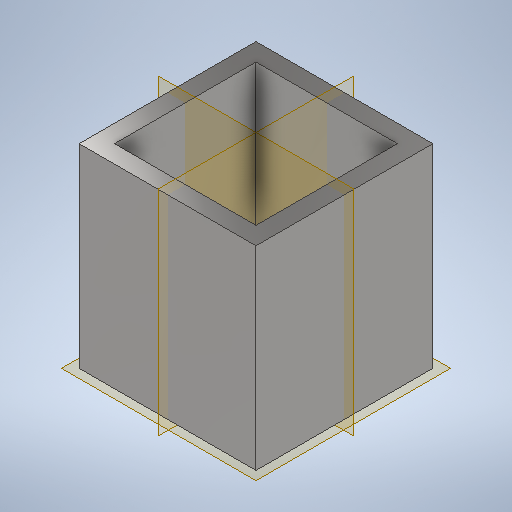
# Autodesk Inventor part: D1_lenght
Saved by Autodesk Inventor 2025.2 (Build 292293000, 293)
## iProperties
Created: 2025-06-19
Part Number: D1_lenght
Material: Steel, Alloy
Document SubType Name: Modeling
Designer: MSIGAMING
Mass: 3061.08 g
Surface Area: 864 cm^2
Volume: 396 cm^3
Density: 7.73 g/cm^3
Appearance: Semi-Polished
Author: MSIGAMING
Autodesk Inventor part; units mm, degrees
sketch "Sketch1" plane through (0, 0, 0) normal (0, 1, 0) x (-1, 0, 0)
  line L0 (50, -50) -> (-50, -50)
  line L1 (-50, -50) -> (-50, 50)
  line L2 (-50, 50) -> (50, 50)
  line L3 (50, 50) -> (50, -50)
  line L4 (50, -50) -> (-50, 50) construction
  line L5 (-50, -50) -> (50, 50) construction
  line L6 (-40, -40) -> (40, -40)
  line L7 (40, -40) -> (40, 40)
  line L8 (40, 40) -> (-40, 40)
  line L9 (-40, 40) -> (-40, -40)
  line L10 (-40, -40) -> (40, 40) construction
  line L11 (40, -40) -> (-40, 40) construction
  point P0 (0, 0)
  dimension "d0" = 100
  dimension "d1" = 100
  dimension "d2" = 80
  dimension "d3" = 80
  constraints: 24 end point, 4 midpoint, 4 parallel, 2 horizontal, 2 perpendicular
  measures "d0" distance of L1.end L2.end
  measures "d1" distance of L0.end L1.end
  measures "d2" distance of L8.end L7.end
  measures "d3" distance of L7.end L6.end
extrude "Extrusion1" add sketch "Sketch1" along normal blind 110
body "Solid1"
